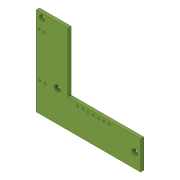
# Autodesk Inventor part: Control Board
Saved by Autodesk Inventor 2017 (Build 210142000, 142)
## iProperties
Created: 2016-08-05
Part Number: Control Board
Material: Generic
Document SubType Name: Modeling
Designer: ge937963
Density: 1 g/cm^3
Appearance: Olive Green
Mass: 1.80659 g
Surface Area: 26.5684 cm^2
Volume: 1.80659 cm^3
Author: ge937963
Autodesk Inventor part; units mm, degrees
ref_plane "YZ Plane" through (0, 0, 0) normal (1, 0, 0) x (0, 1, 0)
ref_plane "XZ Plane" through (0, 0, 0) normal (0, 1, 0) x (-1, 0, 0)
ref_plane "XY Plane" through (0, 0, 0) normal (0, 0, 1) x (1, 0, 0)
sketch "Sketch1" plane through (0, 0, 0) normal (0, 0, 1) x (1, 0, 0)
  line L0 (-25.4, -16.51) -> (25.4, -16.51) projected
  line L1 (25.4, -16.51) -> (25.4, 16.51) projected
  line L2 (25.4, 16.51) -> (-25.4, 16.51) projected
  line L3 (-25.4, 16.51) -> (-25.4, -10.64) projected
  line L4 (-10.0076, 16.51) -> (-10.0076, -12.5222)
  line L5 (-10.0076, -12.5222) -> (25.4, -12.5222)
  line L6 (-25.4, -16.51) -> (-25.4, -26.4922)
  line L7 (-25.4, -26.4922) -> (25.4, -26.4922)
  line L8 (25.4, -26.4922) -> (25.4, -16.51)
  circle A0 centre (-2.54, -13.97) radius 0.5461 projected
  circle A1 centre (2.54, -13.97) radius 0.5461 projected
  circle A2 centre (7.62, -13.97) radius 0.5461 projected
  circle A3 centre (-5.08, -7.62) radius 0.4445 projected
  circle A4 centre (0, -7.62) radius 0.4445 projected
  circle A5 centre (5.08, -7.62) radius 0.4445 projected
  circle A6 centre (10.16, -7.62) radius 0.4445 projected
  circle A7 centre (-5.08, 10.16) radius 0.4445 projected
  circle A8 centre (0, 10.16) radius 0.4445 projected
  circle A9 centre (5.08, 10.16) radius 0.4445 projected
  circle A10 centre (10.16, 10.16) radius 0.4445 projected
  circle A11 centre (12.7, 10.16) radius 0.4445 projected
  circle A12 centre (7.62, 10.16) radius 0.4445 projected
  circle A13 centre (2.54, 10.16) radius 0.4445 projected
  circle A14 centre (-2.54, 10.16) radius 0.4445 projected
  circle A15 centre (12.7, -7.62) radius 0.4445 projected
  circle A16 centre (7.62, -7.62) radius 0.4445 projected
  circle A17 centre (2.54, -7.62) radius 0.4445 projected
  circle A18 centre (-2.54, -7.62) radius 0.4445 projected
  circle A19 centre (10.16, -13.97) radius 0.5461 projected
  circle A20 centre (5.08, -13.97) radius 0.5461 projected
  circle A21 centre (0, -13.97) radius 0.5461 projected
  circle A22 centre (-5.08, -13.97) radius 0.5461 projected
  circle A23 centre (2.6924, -2.0574) radius 0.4445 projected
  circle A24 centre (-2.3876, -2.0574) radius 0.4445 projected
  circle A25 centre (-9.0424, 12.2174) radius 0.4445 projected
  circle A26 centre (-14.1224, 12.2174) radius 0.4445 projected
  circle A27 centre (-16.6624, 12.2174) radius 0.4445 projected
  circle A28 centre (-11.5824, 12.2174) radius 0.4445 projected
  circle A29 centre (-4.9276, -2.0574) radius 0.4445 projected
  circle A30 centre (0.1524, -2.0574) radius 0.4445 projected
  line L9 (-19.25, -14.29) -> (-25.4, -14.29) projected
  line L10 (-25.4, -14.29) -> (-25.4, -16.51) projected
  line L11 (-25.4, -10.64) -> (-19.25, -10.64) projected
  line L12 (-19.25, -10.64) -> (-19.25, -14.29) projected
  line L13 (-25.4, -14.29) -> (-25.4, -10.64)
  line L14 (-25.4, -10.64) -> (-19.25, -10.64)
  line L15 (-19.25, -10.64) -> (-19.25, -14.29)
  line L16 (-19.25, -14.29) -> (-25.4, -14.29)
  circle A31 centre (-23.81, 9.06) radius 0.4445 projected
  circle A32 centre (17.14, 9.37) radius 0.4445 projected
  circle A33 centre (19.68, 9.37) radius 0.4445 projected
  circle A34 centre (-21.27, 9.06) radius 0.4445 projected
  circle A35 centre (19.05, 13.97) radius 1.397 projected
  point P0 (0, 0)
  dimension "d0" = 29.0322
  dimension "d1" = 35.4076
  dimension "d2" = 15.3924
  dimension "d3" = 13.97
  constraints: 18 end point, 3 collinear, 3 perpendicular, 3 vertical, 2 point on line
  measures "d0" distance of L4.start L4.end
  measures "d1" distance of L5.end L4.end
  measures "d2" distance between parallel lines of L3 L4
  measures "d3" distance between parallel lines of L7 L5
extrude "Extrusion1" add sketch "Sketch1" along normal blind 1.6 contours L10 L9 L12 L11 L3 L2 L4 L5 L1 L0 | L0 L8 L7 L6 | L13 L11 L12 L9 | A0 | A1 | A2 | A19 | A20 | A21 | A22 | A26 | A27 | A28 | A31 | A34
sketch "Sketch2" plane through (0, 0, 1.6) normal (0, 0, 1) x (1, 0, 0)
  circle A0 centre (10.16, -13.97) radius 0.5461
  circle A1 centre (7.62, -13.97) radius 0.5461
  circle A2 centre (5.08, -13.97) radius 0.5461
  circle A3 centre (2.54, -13.97) radius 0.5461
  circle A4 centre (0, -13.97) radius 0.5461
  circle A5 centre (-2.54, -13.97) radius 0.5461
  circle A6 centre (-5.08, -13.97) radius 0.5461
  point P0 (0, 0)
extrude "Extrusion2" cut sketch "Sketch2" against normal blind 1.6
sketch "Sketch3" plane through (0, 0, 1.6) normal (0, 0, 1) x (1, 0, 0)
  line L0 (-25.4, 16.51) -> (-25.4, -26.4922) construction
  line L1 (-25.4, 12.11) -> (-10.0076, 12.11) construction
  line L2 (-10.0076, -12.5222) -> (-10.0076, 16.51) construction
  line L3 (-10.0076, 16.51) -> (-25.4, 16.51) construction
  line L4 (25.4, -12.5222) -> (-10.0076, -12.5222) construction
  line L5 (20.07, -12.5222) -> (20.07, -26.4922) construction
  line L6 (-25.4, -26.4922) -> (25.4, -26.4922) construction
  line L7 (25.4, -26.4922) -> (25.4, -12.5222) construction
  point P0 (0, 0)
  dimension "d8" = 4.4
  dimension "d9" = 5.33
  constraints: 4 end point, 4 point on line, 1 horizontal, 1 other
  measures "d8" distance between parallel lines of L3 L1
  measures "d9" distance between parallel lines of L5 L7
sketch "Sketch4" plane through (0, 0, 1.6) normal (0, 0, 1) x (1, 0, 0)
  circle A0 centre (-23.49, -12.3622) radius 0.4445
  circle A1 centre (-20.95, -12.3622) radius 0.4445
  line L0 (-25.4, 16.51) -> (-25.4, -26.4922) projected
  line L1 (-25.4, -26.4922) -> (25.4, -26.4922) projected
  point P0 (0, 0)
  dimension "d10" = 0.889
  dimension "d11" = 0.889
  dimension "d12" = 1.91
  dimension "d13" = 2.54
  dimension "d14" = 0
  dimension "d15" = 14.13
  constraints: 2 centre point
  measures "d10" diameter of A0
  measures "d11" diameter of A1
  measures "d12" distance from line of L0 A0.centre
  measures "d13" distance of A0.centre A1.centre
  measures "d14" vertical distance of A0.centre A1.centre
  measures "d15" distance from line of L1 A0.centre
extrude "Extrusion3" cut sketch "Sketch4" against normal blind 25.4
sketch "Sketch5" plane through (0, 0, 1.6) normal (0, 0, 1) x (1, 0, 0)
  circle A0 centre (-23.81, 9.06) radius 0.4445 projected
  circle A1 centre (17.14, 9.37) radius 0.4445 projected
  circle A2 centre (19.68, 9.37) radius 0.4445 projected
  circle A3 centre (-21.27, 9.06) radius 0.4445 projected
  line L0 (-25.4, -14.29) -> (-19.25, -14.29) projected
  line L1 (-19.25, -14.29) -> (-19.25, -10.64) projected
  line L2 (-19.25, -10.64) -> (-25.4, -10.64) projected
  line L3 (-25.4, 16.51) -> (-25.4, -10.64) projected
  line L4 (25.4, 16.51) -> (-25.4, 16.51) projected
  line L5 (25.4, -16.51) -> (25.4, 16.51) projected
  line L6 (-25.4, -16.51) -> (25.4, -16.51) projected
  line L7 (-25.4, -14.29) -> (-25.4, -16.51) projected
  circle A4 centre (-5.08, -13.97) radius 0.5461 projected
  circle A5 centre (0, -13.97) radius 0.5461 projected
  circle A6 centre (5.08, -13.97) radius 0.5461 projected
  circle A7 centre (10.16, -13.97) radius 0.5461 projected
  circle A8 centre (0.1524, -2.0574) radius 0.4445 projected
  circle A9 centre (-4.9276, -2.0574) radius 0.4445 projected
  circle A10 centre (-11.5824, 12.2174) radius 0.4445 projected
  circle A11 centre (-16.6624, 12.2174) radius 0.4445 projected
  circle A12 centre (-2.54, -7.62) radius 0.4445 projected
  circle A13 centre (2.54, -7.62) radius 0.4445 projected
  circle A14 centre (7.62, -7.62) radius 0.4445 projected
  circle A15 centre (12.7, -7.62) radius 0.4445 projected
  circle A16 centre (-2.54, 10.16) radius 0.4445 projected
  circle A17 centre (2.54, 10.16) radius 0.4445 projected
  circle A18 centre (7.62, 10.16) radius 0.4445 projected
  circle A19 centre (12.7, 10.16) radius 0.4445 projected
  circle A20 centre (10.16, 10.16) radius 0.4445 projected
  circle A21 centre (5.08, 10.16) radius 0.4445 projected
  circle A22 centre (0, 10.16) radius 0.4445 projected
  circle A23 centre (-5.08, 10.16) radius 0.4445 projected
  circle A24 centre (10.16, -7.62) radius 0.4445 projected
  circle A25 centre (5.08, -7.62) radius 0.4445 projected
  circle A26 centre (0, -7.62) radius 0.4445 projected
  circle A27 centre (-5.08, -7.62) radius 0.4445 projected
  circle A28 centre (-14.1224, 12.2174) radius 0.4445 projected
  circle A29 centre (-9.0424, 12.2174) radius 0.4445 projected
  circle A30 centre (-2.3876, -2.0574) radius 0.4445 projected
  circle A31 centre (2.6924, -2.0574) radius 0.4445 projected
  circle A32 centre (7.62, -13.97) radius 0.5461 projected
  circle A33 centre (2.54, -13.97) radius 0.5461 projected
  circle A34 centre (-2.54, -13.97) radius 0.5461 projected
  circle A35 centre (19.05, 13.97) radius 1.397 projected
  point P0 (0, 0)
extrude "Extrusion4" cut sketch "Sketch5" against normal blind 25.4 contours A0 | A3
sketch "Sketch6" plane through (0, 0, 1.6) normal (0, 0, 1) x (1, 0, 0)
  circle A0 centre (22.7674, -19.4372) radius 1.397
  point P0 (0, 0)
  dimension "d20" = 2.794
  constraints: 1 centre point
  measures "d20" diameter of A0
extrude "Extrusion5" cut sketch "Sketch6" against normal blind 25.4
sketch "Sketch7" plane through (0, 0, 0) normal (0, 0, -1) x (-1, 0, 0)
  circle A0 centre (15.0353, -11.3709) radius 1.397
  line L0 (24.1179, -7.9159) -> (10.0987, -7.9159) projected
  point P0 (0, 0)
  dimension "d23" = 2.794
  dimension "d24" = 3.455
  constraints: 1 centre point
  measures "d23" diameter of A0
  measures "d24" distance from line of A0.centre L0
extrude "Extrusion6" cut sketch "Sketch7" against normal blind 25.4
sketch "Sketch8" plane through (0, 0, 1.6) normal (0, 0, 1) x (1, 0, 0)
  circle A0 centre (-22.4387, 14.4799) radius 1.397
  point P0 (0, 0)
  dimension "d27" = 2.794
  constraints: 1 centre point
  measures "d27" diameter of A0
extrude "Extrusion7" cut sketch "Sketch8" against normal blind 25.4
body "Solid1"
